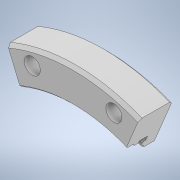
# Autodesk Inventor part: prueba_clamp_iso160
Saved by Autodesk Inventor 2021 (Build 250183000, 183)
## iProperties
Created: 2024-01-17
Part Number: prueba_clamp_iso160
Material: Generic
Document SubType Name: Modeling
Designer: Sebastián
Density: 1 g/cm^3
Appearance: Default
Author: Sebastián
Autodesk Inventor part; units mm, degrees
ref_plane "YZ Plane" through (0, 0, 0) normal (1, 0, 0) x (0, 1, 0)
ref_plane "XZ Plane" through (0, 0, 0) normal (0, 1, 0) x (-1, 0, 0)
ref_plane "XY Plane" through (0, 0, 0) normal (0, 0, 1) x (1, 0, 0)
sketch "Sketch1" plane through (0, 0, 0) normal (1, 0, 0) x (0, 1, 0)
  line L0 (81.2, 2.1737) -> (83.2, 2.1737)
  line L1 (83.2, 2.1737) -> (83.2, 4.1737)
  line L2 (83.2, 4.1737) -> (87.2, 4.1737)
  line L3 (87.2, 4.1737) -> (87.2, 2.1737)
  line L4 (87.2, 2.1737) -> (90.2, 2.1737)
  line L5 (90.2, 2.1737) -> (90.2, 7.1737)
  arc A0 (90.2, 11.1737) -> (90.2, 7.1737) centre (90.2, 9.1737) ccw
  line L6 (90.2, 11.1737) -> (90.2, 16.1737)
  line L7 (90.2, 16.1737) -> (92.2, 16.1737)
  line L8 (92.2, 16.1737) -> (92.2, 16.1737)
  line L9 (92.2, 16.1737) -> (112.2, 16.1737)
  line L10 (112.2, 16.1737) -> (112.2, -5.8263)
  line L11 (112.2, -5.8263) -> (81.2, -5.8263)
  line L12 (81.2, -5.8263) -> (81.2, 2.1737)
  line L13 (90.2, 11.1737) -> (90.2, 7.1737) construction
  line L14 (0, -10.2263) -> (0, 20.5737) projected
  point P0 (0, 0)
  dimension "d0" = 4
  dimension "d1" = 9
  dimension "d2" = 3
  dimension "d3" = 2
  dimension "d4" = 5
  dimension "d5" = 4
  dimension "d6" = 90.2
  dimension "d8" = 20
  dimension "d9" = 2
  dimension "d21" = 81.2
  dimension "d22" = 8
  dimension "d23" = 14
  dimension "d25" = 22
  dimension "d40" = 0
  constraints: 28 end point, 10 perpendicular, 2 point on circle, 2 point on line, 2 vertical, 1 centre point, 1 coincident, 1 horizontal, 1 midpoint
  measures "d0" distance of L1.end L2.end
  measures "d1" distance of L0.start L4.end
  measures "d2" distance of L4.end L3.end
  measures "d3" distance of L0.end L1.end
  measures "d4" distance of L4.end L5.end
  measures "d5" distance of L5.end L6.start
  measures "d6" horizontal distance of point (0, 0) L4.end
  measures "d8" distance of L8.end L9.end
  measures "d9" distance of L7.end L6.end
  measures "d21" horizontal distance of point (0, 0) L0.start
  measures "d22" distance of L11.end L0.start
  measures "d23" distance of L6.end L4.end
  measures "d25" distance of L9.end L10.end
  measures "d40" vertical distance of L6.end L8.end
revolve "Revolution1" add sketch "Sketch1" angle 45 mid plane about axis through (0, 0, -10) along (0, 0, 1)
chamfer "Chamfer2" distance 1 angle 45 4 edges at (0, 83.2, 4.1737) (0, 87.2, 4.1737) (0, 81.2, 2.1737) (0, 90.2, 16.1737)
chamfer "Chamfer3" distance 2 angle 45 2 edges at (0, 112.2, -5.8263) (0, 112.2, 16.1737)
sketch "Sketch5" plane through (0, 0, 16.1737) normal (0, 0, 1) x (1, 0, 0)
  circle A0 centre (26.6584, 99.4904) radius 5.25
  circle A1 centre (-26.6584, 99.4904) radius 5.25
  arc A2 (-1.1976, 102.993) -> (-50.3773, 89.8395) centre (0, 0) ccw construction
  line L0 (0, 0) -> (-26.6584, 99.4904) construction
  line L1 (0, -22.44) -> (0, 134.64) construction
  dimension "d41" = 103
  dimension "d42" = 10.5
  dimension "d43" = 15
  constraints: 3 centre point, 3 point on circle, 2 end point, 1 coincident, 1 equal radius, 1 symmetric about line
  measures "d41" radius of A2
  measures "d42" diameter of A0
  measures "d43" angle of L1 L0
extrude "Extrusion4" cut sketch "Sketch5" against normal through all
body "Solid1"
